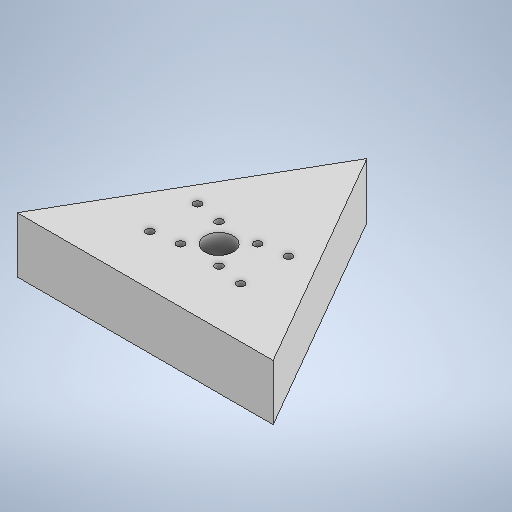
# Autodesk Inventor part: SupportingMainBracket
Saved by Autodesk Inventor 2027 (Build 310192060, 192F)
## iProperties
Created: 2026-07-10
Part Number: SupportingMainBracket
Material: Generic
Document SubType Name: Modeling
Designer: 13129
Density: 1 g/cm^3
Appearance: Default
Author: 13129
Autodesk Inventor part; units mm, degrees
ref_plane "YZ Plane" through (0, 0, 0) normal (1, 0, 0) x (0, 1, 0)
ref_plane "XZ Plane" through (0, 0, 0) normal (0, 1, 0) x (-1, 0, 0)
ref_plane "XY Plane" through (0, 0, 0) normal (0, 0, 1) x (1, 0, 0)
sketch "Sketch1" plane through (0, 0, 0) normal (0, 1, 0) x (-1, 0, 0)
  line L0 (0, -58.7743) -> (-50.9, 29.3871)
  line L1 (-50.9, 29.3871) -> (50.9, 29.3871)
  line L2 (50.9, 29.3871) -> (0, -58.7743)
  line L3 (0, -65.1243) -> (-56.3993, 32.5621)
  line L4 (-56.3993, 32.5621) -> (56.3993, 32.5621)
  line L5 (56.3993, 32.5621) -> (0, -65.1243)
  line L6 (-13.2848, -35.7643) -> (0, -28.0943)
  line L7 (0, -28.0943) -> (13.2848, -35.7643)
  line L8 (37.6152, 6.3771) -> (24.3303, 14.0471)
  line L9 (24.3303, 14.0471) -> (24.3303, 29.3871)
  line L10 (-24.3303, 29.3871) -> (-24.3303, 14.0471)
  line L11 (-24.3303, 14.0471) -> (-37.6152, 6.3771)
  point P0 (0, 0)
  point P1 (0, 0)
  point P2 (0, 0)
  dimension "d0" = 101.8
  dimension "d3" = 6.35
  dimension "d4" = 30.68
  dimension "d7" = 360
  constraints: 24 end point, 3 vertical alignment, 2 coincident, 2 perpendicular, 2 point on line, 30 other
  measures "d0" distance of L0.end L1.end
  measures "d3" distance of L3.start L0.start
  measures "d4" distance of L6.end L0.start
extrude "Extrusion1" add sketch "Sketch1" along normal blind 12.5 contours L0 L11 L10 L1 L9 L8 L2 L7 L6 | L3 L4 L5
sketch "Sketch3" plane through (0, 12.5, 0) normal (0, 1, 0) x (1, 0, 0)
  line L0 (0, 65.1243) -> (56.3993, -32.5621)
  line L1 (56.3993, -32.5621) -> (-56.3993, -32.5621)
  line L2 (-56.3993, -32.5621) -> (0, 65.1243)
  point P0 (0, 0)
  point P1 (0, 0)
  constraints: 6 end point, 1 coincident, 7 other
extrude "Extrusion2" add sketch "Sketch3" along normal blind 12
sketch "Sketch4" plane through (0, 24.5, 0) normal (0, 1, 0) x (1, 0, 0)
  line L0 (-56.3993, -32.5621) -> (56.3993, -32.5621) construction
  line L1 (56.3993, -32.5621) -> (0, 65.1243) construction
  line L2 (-23.5, -13.7189) -> (23.5, -13.7189)
  line L3 (23.5, -13.7189) -> (23.5, 16.2811)
  line L4 (23.5, 16.2811) -> (-23.5, 16.2811)
  line L5 (-23.5, 16.2811) -> (-23.5, -13.7189)
  circle A0 centre (0, 0) radius 6.25
  circle A1 centre (-8.5, 8.5) radius 1.7
  circle A2 centre (-20, 10.5) radius 1.7
  circle A3 centre (8.5, 8.5) radius 1.7
  circle A4 centre (20, 10.5) radius 1.7
  circle A5 centre (8.5, -8.5) radius 1.7
  circle A6 centre (20, -10.5) radius 1.7
  circle A7 centre (-8.5, -8.5) radius 1.7
  circle A8 centre (-20, -10.5) radius 1.7
  line L6 (-20, 10.5) -> (20, 10.5) construction
  line L7 (20, 10.5) -> (20, -10.5) construction
  line L8 (-8.5, 8.5) -> (8.5, 8.5) construction
  line L9 (8.5, 8.5) -> (8.5, -8.5) construction
  point P0 (28.1996, 16.2811)
  point P1 (0, -13.7189)
  point P2 (0, -32.5621)
  point P3 (8.5, 0)
  point P4 (20, 0)
  point P5 (0, 8.5)
  point P6 (0, 10.5)
  dimension "d11" = 47
  dimension "d12" = 30
  dimension "d13" = 12.5
  dimension "d14" = 3.4
  dimension "d15" = 40
  dimension "d16" = 17
  dimension "d17" = 21
  dimension "d18" = 17
  constraints: 16 end point, 9 centre point, 7 equal radius, 7 horizontal alignment, 7 midpoint, 7 vertical alignment, 4 horizontal, 4 perpendicular, 1 coincident
  measures "d11" distance of L2.start L2.end
  measures "d12" distance of L2.end L3.end
  measures "d13" diameter of A0
  measures "d14" diameter of A2
  measures "d15" distance of L6.start L6.end
  measures "d16" distance of L8.end L9.end
  measures "d17" distance of L6.end L7.end
  measures "d18" distance of L8.start L8.end
extrude "Extrusion3" cut sketch "Sketch4" along normal through all both and the other way through all contours A0 | A1 | A2 | A3 | A4 | A5 | A6 | A7 | A8
sketch "Sketch5" plane through (0, 0, 0) normal (0, -1, 0) x (1, 0, 0)
  line L0 (-56.3993, 32.5621) -> (56.3993, 32.5621) construction
  line L1 (8.382, 24.9421) -> (-8.382, 24.9421) construction
  line L2 (-8.382, 24.9421) -> (-8.382, 31.2921) construction
  line L3 (-8.382, 31.2921) -> (8.382, 31.2921) construction
  line L4 (8.382, 31.2921) -> (8.382, 24.9421) construction
  spline S0 degree 2 poles (8.287, 30.3523) (8.7545, 30.92) (9.1839, 31.1251) knots 0 0 0 1 1 1
  spline S1 degree 2 poles (9.1839, 31.1251) (9.6467, 31.3589) (10.2716, 31.3589) knots 0 0 0 1 1 1
  spline S2 degree 2 poles (10.2716, 31.3589) (11.3308, 31.3589) (12.7, 29.5651) (12.7, 28.0909) knots 0 0 0 1 2 2 2
  spline S3 degree 2 poles (12.7, 28.0909) (12.7, 26.4831) (11.7745, 25.6053) knots 0 0 0 1 1 1
  spline S4 degree 2 poles (11.7745, 25.6053) (11.2974, 24.9421) (10.4052, 24.9421) knots 0 0 0 1 1 1
  spline S5 degree 2 poles (10.4052, 24.9421) (9.7039, 24.9421) (9.2554, 25.1759) knots 0 0 0 1 1 1
  spline S6 degree 2 poles (9.2554, 25.1759) (8.8642, 25.3667) (8.5398, 25.9297) knots 0 0 0 1 1 1
  spline S7 degree 2 poles (8.5398, 25.9297) (8.4778, 26.0299) (8.4778, 26.1253) knots 0 0 0 1 1 1
  spline S8 degree 2 poles (8.4778, 26.1253) (8.4778, 26.2684) (8.702, 26.4831) (8.8595, 26.4831) knots 0 0 0 1 2 2 2
  spline S9 degree 2 poles (8.8595, 26.4831) (9.0551, 26.4831) (9.1743, 26.278) knots 0 0 0 1 1 1
  spline S10 degree 2 poles (9.1743, 26.278) (9.3699, 25.944) (9.6323, 25.8104) knots 0 0 0 1 1 1
  spline S11 degree 2 poles (9.6323, 25.8104) (9.9281, 25.6864) (10.41, 25.6864) knots 0 0 0 1 1 1
  spline S12 degree 2 poles (10.41, 25.6864) (11.0254, 25.6864) (11.4453, 26.2064) knots 0 0 0 1 1 1
  spline S13 degree 2 poles (11.4453, 26.2064) (11.9701, 26.8505) (11.9701, 28.0909) knots 0 0 0 1 1 1
  spline S14 degree 2 poles (11.9701, 28.0909) (11.9701, 29.2216) (10.9873, 30.6242) (10.2573, 30.6242) knots 0 0 0 1 2 2 2
  spline S15 degree 2 poles (10.2573, 30.6242) (9.4511, 30.6242) (8.8499, 29.8895) knots 0 0 0 1 1 1
  spline S16 degree 2 poles (8.8499, 29.8895) (8.7402, 29.7559) (8.5828, 29.7559) knots 0 0 0 1 1 1
  spline S17 degree 2 poles (8.5828, 29.7559) (8.4349, 29.7559) (8.2106, 29.9801) (8.2106, 30.1233) knots 0 0 0 1 2 2 2
  spline S18 degree 2 poles (8.2106, 30.1233) (8.2106, 30.2521) (8.287, 30.3523) knots 0 0 0 1 1 1
  line L5 (4.4989, 29.0594) -> (6.7221, 29.0594)
  spline S19 degree 2 poles (6.7221, 29.0594) (7.0895, 29.0594) (7.0895, 28.692) knots 0 0 0 1 1 1
  spline S20 degree 2 poles (7.0895, 28.692) (7.0895, 28.3342) (6.7221, 28.3342) knots 0 0 0 1 1 1
  line L6 (6.7221, 28.3342) -> (4.4989, 28.3342)
  spline S21 degree 2 poles (4.4989, 28.3342) (4.1268, 28.3342) (4.1268, 28.692) knots 0 0 0 1 1 1
  spline S22 degree 2 poles (4.1268, 28.692) (4.1268, 29.0594) (4.4989, 29.0594) knots 0 0 0 1 1 1
  line L7 (-0.916, 25.4574) -> (0.6775, 31.0297)
  spline S23 degree 2 poles (0.6775, 31.0297) (0.7681, 31.3351) (1.1545, 31.3351) knots 0 0 0 1 1 1
  spline S24 degree 2 poles (1.1545, 31.3351) (1.541, 31.3351) (1.6459, 30.9343) knots 0 0 0 1 1 1
  line L8 (1.6459, 30.9343) -> (3.4302, 25.4717)
  spline S25 degree 2 poles (3.4302, 25.4717) (3.4541, 25.4049) (3.4541, 25.3429) knots 0 0 0 1 1 1
  spline S26 degree 2 poles (3.4541, 25.3429) (3.4541, 24.9946) (3.0867, 24.9946) knots 0 0 0 1 1 1
  spline S27 degree 2 poles (3.0867, 24.9946) (2.8339, 24.9946) (2.8148, 25.1854) knots 0 0 0 1 1 1
  line L9 (2.8148, 25.1854) -> (1.1641, 30.2664)
  line L10 (1.1641, 30.2664) -> (-0.2195, 25.2475)
  spline S28 degree 2 poles (-0.2195, 25.2475) (-0.291, 24.9946) (-0.5486, 24.9946) knots 0 0 0 1 1 1
  spline S29 degree 2 poles (-0.5486, 24.9946) (-0.6918, 24.9946) (-0.9303, 25.1998) (-0.9303, 25.3524) knots 0 0 0 1 2 2 2
  spline S30 degree 2 poles (-0.9303, 25.3524) (-0.9303, 25.3954) (-0.916, 25.4574) knots 0 0 0 1 1 1
  spline S31 degree 2 poles (-6.9941, 30.8294) (-7.0322, 30.9009) (-7.0322, 30.982) knots 0 0 0 1 1 1
  spline S32 degree 2 poles (-7.0322, 30.982) (-7.0322, 31.3351) (-6.6506, 31.3351) knots 0 0 0 1 1 1
  spline S33 degree 2 poles (-6.6506, 31.3351) (-6.412, 31.3351) (-6.3166, 31.0965) knots 0 0 0 1 1 1
  line L11 (-6.3166, 31.0965) -> (-5.9349, 30.1424)
  line L12 (-5.9349, 30.1424) -> (-2.8577, 30.1424)
  line L13 (-2.8577, 30.1424) -> (-2.4856, 31.0965)
  spline S34 degree 2 poles (-2.4856, 31.0965) (-2.395, 31.3351) (-2.1469, 31.3351) knots 0 0 0 1 1 1
  spline S35 degree 2 poles (-2.1469, 31.3351) (-1.7795, 31.3351) (-1.7795, 30.9773) knots 0 0 0 1 1 1
  spline S36 degree 2 poles (-1.7795, 30.9773) (-1.7795, 30.9057) (-1.7986, 30.8484) knots 0 0 0 1 1 1
  line L14 (-1.7986, 30.8484) -> (-3.9264, 25.1854)
  spline S37 degree 2 poles (-3.9264, 25.1854) (-4.0171, 24.9421) (-4.351, 24.9421) knots 0 0 0 1 1 1
  spline S38 degree 2 poles (-4.351, 24.9421) (-4.6897, 24.9421) (-4.7756, 25.1759) knots 0 0 0 1 1 1
  line L15 (-4.7756, 25.1759) -> (-6.9941, 30.8294)
  line L16 (-5.6916, 29.3981) -> (-4.351, 25.944)
  line L17 (-4.351, 25.944) -> (-3.0963, 29.3981)
  line L18 (-3.0963, 29.3981) -> (-5.6916, 29.3981)
  spline S39 degree 2 poles (-12.4185, 30.9677) (-12.4185, 31.3255) (-12.1084, 31.3255) knots 0 0 0 1 1 1
  spline S40 degree 2 poles (-12.1084, 31.3255) (-11.889, 31.3255) (-11.7172, 31.0822) knots 0 0 0 1 1 1
  line L19 (-11.7172, 31.0822) -> (-8.5255, 26.2684)
  line L20 (-8.5255, 26.2684) -> (-8.5255, 30.9486)
  spline S41 degree 2 poles (-8.5255, 30.9486) (-8.5255, 31.3255) (-8.1534, 31.3255) knots 0 0 0 1 1 1
  spline S42 degree 2 poles (-8.1534, 31.3255) (-7.786, 31.3255) (-7.786, 30.9486) knots 0 0 0 1 1 1
  line L21 (-7.786, 30.9486) -> (-7.786, 25.3238)
  spline S43 degree 2 poles (-7.786, 25.3238) (-7.786, 24.9755) (-8.12, 24.9755) knots 0 0 0 1 1 1
  spline S44 degree 2 poles (-8.12, 24.9755) (-8.3585, 24.9755) (-8.5255, 25.2188) knots 0 0 0 1 1 1
  line L22 (-8.5255, 25.2188) -> (-11.6886, 29.9515)
  line L23 (-11.6886, 29.9515) -> (-11.6886, 25.3524)
  spline S45 degree 2 poles (-11.6886, 25.3524) (-11.6886, 24.9755) (-12.0559, 24.9755) knots 0 0 0 1 1 1
  spline S46 degree 2 poles (-12.0559, 24.9755) (-12.4185, 24.9755) (-12.4185, 25.3524) knots 0 0 0 1 1 1
  line L24 (-12.4185, 25.3524) -> (-12.4185, 30.9677)
  point P0 (0, 31.2921)
  point P1 (0, 32.5621)
  dimension "d21" = 6.35
  dimension "d22" = 16.764
  dimension "d28" = 1.27
  constraints: 2 midpoint, 1 vertical alignment, 2 other
  measures "d21" distance of L3.end L1.start
  measures "d22" distance of L1.start L1.end
  measures "d28" distance between parallel lines of L3 L0
extrude "Extrusion4" add sketch "Sketch5" along normal blind 1
pattern_circular "Circular Pattern1" count 3 over 360 about axis through (0, -10, 0) along (0, 1, 0) of "Extrusion4"
body "Solid1"
